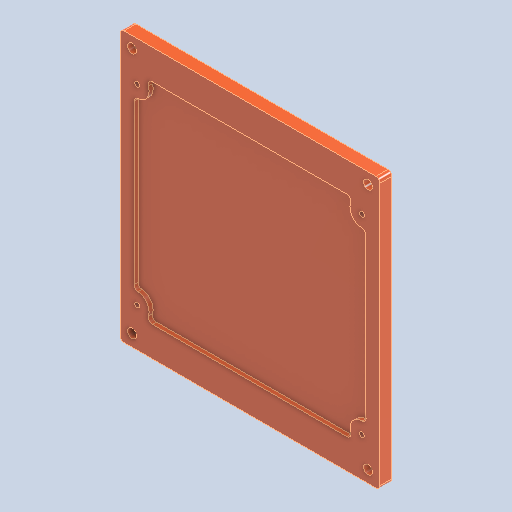
# Autodesk Inventor part: chapa da pcb
Saved by Autodesk Inventor 2026 (Build 300175050, 175E)
## iProperties
Created: 2025-07-31
Part Number: chapa da pcb
Material: Genérico
Document SubType Name: Modeling
Designer: Kedso
Density: 1 g/cm^3
Appearance: Suave - Laranja claro
Author: Kedson Neves
Autodesk Inventor part; units mm, degrees
ref_plane "YZ Plane" through (0, 0, 0) normal (1, 0, 0) x (0, 1, 0)
ref_plane "XZ Plane" through (0, 0, 0) normal (0, 1, 0) x (-1, 0, 0)
ref_plane "XY Plane" through (0, 0, 0) normal (0, 0, 1) x (1, 0, 0)
sketch "Esboço1" plane through (0, 0, 0) normal (0, 0, 1) x (1, 0, 0)
  line L0 (60.7325, -52.1672) -> (60.7325, 51.7628)
  line L1 (-60.7775, 51.7628) -> (-60.7775, -52.1672)
  line L2 (60.7325, -0.2022) -> (-60.7775, -0.2022)
  line L3 (64.9775, 67.2978) -> (-65.0225, 67.2978)
  line L4 (-65.0225, 67.2978) -> (-65.0225, -67.7022)
  line L5 (-65.0225, -67.7022) -> (64.9775, -67.7022)
  line L6 (64.9775, -67.7022) -> (64.9775, 67.2978)
  line L7 (64.9775, 67.2978) -> (-65.0225, -67.7022) construction
  line L8 (-65.0225, 67.2978) -> (64.9775, -67.7022) construction
  circle A0 centre (55.9625, -48.1472) radius 1.8
  circle A1 centre (55.9625, 47.3828) radius 1.8
  circle A2 centre (-56.4575, 47.3828) radius 1.8
  circle A3 centre (-56.4575, -48.1472) radius 1.8
  circle A4 centre (-56.4575, 47.3828) radius 0.7501
  circle A5 centre (-56.4575, -48.1472) radius 1.059
  circle A6 centre (55.9625, -48.1472) radius 0.7793
  circle A7 centre (55.9625, 47.3828) radius 0.9848
  point P0 (0, 0)
  point P1 (-0.0225, -0.2022)
  dimension "d0" = 135
  dimension "d1" = 130
  constraints: 18 end point, 8 centre point, 5 midpoint, 2 parallel, 1 horizontal, 1 perpendicular
  measures "d0" distance of L5.end L3.start
  measures "d1" distance of L4.end L5.end
extrude "Extrusão1" add sketch "Esboço1" along normal blind 6 contours L6 L5 L4 L3 | A0 | A1 | A2 | A3
sketch "Esboço2" plane through (0, 0, 6) normal (0, 0, 1) x (1, 0, 0)
  circle A0 centre (-56.4575, 47.3828) radius 0.7501 projected
  circle A1 centre (55.9625, 47.3828) radius 0.9848 projected
  circle A2 centre (55.9625, -48.1472) radius 0.7793 projected
  circle A3 centre (-56.4575, -48.1472) radius 1.059 projected
  point P0 (0, 0)
  constraints: 4 coincident
hole "Furo1" at (-56.4575, 47.3828, 6) at (55.9625, 47.3828, 6) at (55.9625, -48.1472, 6) at (-56.4575, -48.1472, 6) direction (0, 0, -1) diameter 2.459 end through all thread size "M3x0.5" class "6H" standard "ISO Metric profile"
sketch "Esboço3" plane through (0, 0, 6) normal (0, 0, 1) x (1, 0, 0)
  line L0 (64.9775, 67.2978) -> (-65.0225, 67.2978) projected
  line L1 (-0.0225, 67.2978) -> (-0.0225, -67.7022)
  line L2 (-65.0225, -67.7022) -> (64.9775, -67.7022) projected
  line L3 (-58.0225, -52.7022) -> (57.9775, -52.7022)
  line L4 (57.9775, -52.7022) -> (57.9775, 52.2978)
  line L5 (57.9775, 52.2978) -> (-58.0225, 52.2978)
  line L6 (-58.0225, 52.2978) -> (-58.0225, -52.7022)
  line L7 (-58.0225, -52.7022) -> (57.9775, 52.2978) construction
  line L8 (57.9775, -52.7022) -> (-58.0225, 52.2978) construction
  circle A0 centre (-56.4575, 47.3828) radius 1.2295 projected
  circle A1 centre (-56.4575, 47.3828) radius 6
  circle A2 centre (55.9625, 47.3828) radius 1.2295 projected
  circle A3 centre (55.9625, 47.3828) radius 6
  circle A4 centre (-56.4575, -48.1472) radius 1.2295 projected
  circle A5 centre (-56.4575, -48.1472) radius 6
  circle A6 centre (55.9625, -48.1472) radius 1.2295 projected
  circle A7 centre (55.9625, -48.1472) radius 6
  point P0 (-0.0225, -0.2022)
  point P1 (-58.0225, -42.3549)
  point P2 (-52.5521, -52.7022)
  point P3 (52.0572, -52.7022)
  point P4 (57.9775, -42.4957)
  point P5 (57.9775, 41.7313)
  point P6 (52.5212, 52.2978)
  point P7 (-53.0161, 52.2978)
  point P8 (-58.0225, 41.5905)
  dimension "d16" = 116
  dimension "d17" = 105
  dimension "d18" = 12
  constraints: 14 end point, 5 midpoint, 4 centre point, 4 coincident, 3 equal radius, 2 parallel, 1 horizontal, 1 perpendicular
  measures "d16" distance of L4.end L5.end
  measures "d17" distance of L5.end L3.start
  measures "d18" diameter of A1
extrude "Extrusão2" cut sketch "Esboço3" against normal blind 2 contours L5 A3 L4 A7 L3 L1 | L1 L3 A5 L6 A1 L5
fillet "Arredondamento1" radius 2 8 edges at (-58.0225, -42.3549, 5) (-52.5521, -52.7022, 5) (52.0572, -52.7022, 5) (57.9775, -42.4957, 5) (57.9775, 41.7313, 5) (52.5212, 52.2978, 5) (-53.0161, 52.2978, 5) (-58.0225, 41.5905, 5)
sketch "Esboço4" plane through (0, 0, 6) normal (0, 0, 1) x (1, 0, 0)
  line L0 (0, 0) -> (0, -87.1961)
  line L1 (0, 0) -> (-82.4398, 0)
  line L2 (-65.0225, -67.7022) -> (64.9775, -67.7022) projected
  line L3 (-65.0225, 67.2978) -> (-65.0225, -67.7022) projected
  line L4 (-65.0225, 67.7022) -> (64.9775, 67.7022)
  point P0 (-59.0225, -61.7022)
  point P1 (59.0225, -61.7022)
  point P2 (65.0225, -67.7022)
  point P3 (-59.0225, 61.7022)
  point P4 (65.0225, 67.7022)
  point P5 (59.0225, 61.7022)
  dimension "d22" = 6
  dimension "d23" = 6
  constraints: 7 symmetric about line, 6 end point, 1 horizontal, 1 vertical
  measures "d22" distance from line of L2 point (-59.022, -61.702)
  measures "d23" distance from line of L3 point (-59.022, -61.702)
hole "Furo2" at (-59.0225, -61.7022, 6) at (59.0225, -61.7022, 6) at (59.0225, 61.7022, 6) at (-59.0225, 61.7022, 6) direction (0, 0, -1) diameter 4.5 end through all
fillet "Arredondamento2" radius 2 4 edges at (64.9775, -67.7022, 3) (-65.0225, -67.7022, 3) (-65.0225, 67.2978, 3) (64.9775, 67.2978, 3)
